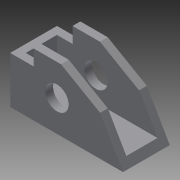
# Autodesk Inventor part: 2.4 Tutorial
Saved by Autodesk Inventor 2015 (Build 190159000, 159)
## iProperties
Created: 2015-09-02
Part Number: 2.4 Tutorial
Material: Generic
Document SubType Name: Modeling
Designer: Brandon
Density: 1 g/cm^3
Appearance: Default
Author: Brandon
Autodesk Inventor part; units mm, degrees
ref_plane "YZ Plane" through (0, 0, 0) normal (1, 0, 0) x (0, 1, 0)
ref_plane "XZ Plane" through (0, 0, 0) normal (0, 1, 0) x (-1, 0, 0)
ref_plane "XY Plane" through (0, 0, 0) normal (0, 0, 1) x (1, 0, 0)
sketch "Sketch1" plane through (0, 0, 0) normal (0, 0, 1) x (1, 0, 0)
  line L0 (0, 0) -> (91.948, 0)
  line L1 (0, 0) -> (0, 38.1)
  line L2 (0, 38.1) -> (19.05, 38.1)
  line L3 (19.05, 38.1) -> (19.05, 50.8)
  line L4 (19.05, 50.8) -> (41.402, 50.8)
  line L5 (91.948, 0) -> (223.0777, 0) construction
  line L6 (41.402, 50.8) -> (73.2269, 32.4259)
  line L7 (91.948, 0) -> (73.2269, 32.4259)
  circle A0 centre (38.1, 25.4) radius 9.525
  dimension "d3" = 12.7
  dimension "d7" = 19.05
  dimension "d8" = 50.8
  dimension "d9" = 41.402
  dimension "d10" = 60
  dimension "d11" = 30
  dimension "d12" = 19.05
  dimension "d13" = 38.1
  dimension "d14" = 25.4
  constraints: 16 end point, 3 perpendicular, 2 horizontal, 1 centre point, 1 vertical
  measures "d3" distance of L2.end L3.end
  measures "d7" distance of L1.end L2.end
  measures "d8" vertical distance of L0.start L3.end
  measures "d9" horizontal distance of L4.end L1.end
  measures "d10" angle of L0 L7
  measures "d11" angle of L7 L6
  measures "d12" diameter of A0
  measures "d13" horizontal distance of L0.start A0.centre
  measures "d14" vertical distance of L0.end A0.centre
extrude "Extrusion1" add sketch "Sketch1" along normal blind 6.35
sketch "Sketch2" plane through (0, 0, 0) normal (0, 0, -1) x (-1, 0, 0)
  line L0 (-19.05, 38.1) -> (0, 38.1) projected
  line L1 (0, 0) -> (-6.35, 0)
  line L2 (-6.35, 0) -> (-6.35, 38.1)
  line L3 (-6.35, 38.1) -> (0, 38.1)
  line L4 (0, 38.1) -> (0, 0)
  dimension "d17" = 6.35
  constraints: 8 end point, 2 parallel, 1 horizontal, 1 perpendicular, 1 point on line
  measures "d17" distance of L2.end L3.end
extrude "Extrusion2" add sketch "Sketch2" along normal blind 25.4
sketch "Sketch3" plane through (0, 0, 0) normal (0, 0, -1) x (-1, 0, 0)
  point P0 (0, 0)
sketch "Sketch4" plane through (0, 0, 0) normal (0, 0, -1) x (-1, 0, 0)
  line L0 (-6.35, 0) -> (-6.35, 6.35)
  line L1 (-6.35, 0) -> (-6.35, 38.1) projected
  line L2 (-6.35, 6.35) -> (-88.2818, 6.35)
  line L3 (-88.2818, 6.35) -> (-91.948, 0)
  line L4 (-91.948, 0) -> (-73.2269, 32.4259) projected
  line L5 (-91.948, 0) -> (-6.35, 0)
  line L6 (0, 0) -> (-91.948, 0) projected
  dimension "d21" = 6.35
  constraints: 8 end point, 2 collinear, 1 perpendicular, 1 point on line
  measures "d21" distance of L0.start L0.end
extrude "Extrusion3" add sketch "Sketch4" along normal blind 25.4
sketch "Sketch5" plane through (0, 0, -25.4) normal (0, 0, -1) x (-1, 0, 0)
  point P0 (0, 0)
sketch "Sketch6" plane through (0, 0, -25.4) normal (0, 0, -1) x (-1, 0, 0)
  line L0 (0, 0) -> (0, 38.1)
  line L1 (0, 38.1) -> (-19.05, 38.1)
  line L2 (-19.05, 38.1) -> (-19.05, 50.8)
  line L3 (-19.05, 50.8) -> (-41.402, 50.8)
  line L4 (-41.402, 50.8) -> (-73.2269, 32.4259)
  line L5 (-73.2269, 32.4259) -> (-91.948, 0)
  line L6 (-91.948, 0) -> (0, 0)
  line L7 (0, 0) -> (-91.948, 0) projected
  circle A0 centre (-38.1, 25.4) radius 9.525
  dimension "d24" = 19.05
  dimension "d25" = 38.1
  dimension "d26" = 25.4
  constraints: 14 end point, 3 perpendicular, 1 centre point, 1 collinear, 1 vertical
  measures "d24" diameter of A0
  measures "d25" distance from line of L0 A0.centre
  measures "d26" vertical distance of L5.end A0.centre
extrude "Extrusion4" add sketch "Sketch6" along normal blind 6.35
body "Solid1"
